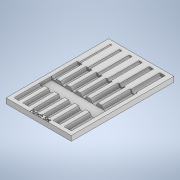
# Autodesk Inventor part: punchTray
Saved by Autodesk Inventor 2020.2 (Build 242310000, 310)
## iProperties
Created: 2019-12-07
Part Number: punchTray
Material: Generic
Document SubType Name: Modeling
Designer: robst
Density: 1 g/cm^3
Appearance: Default
Author: robst
Autodesk Inventor part; units mm, degrees
ref_plane "YZ Plane" through (0, 0, 0) normal (1, 0, 0) x (0, 1, 0)
ref_plane "XZ Plane" through (0, 0, 0) normal (0, 1, 0) x (-1, 0, 0)
ref_plane "XY Plane" through (0, 0, 0) normal (0, 0, 1) x (1, 0, 0)
sketch "Sketch3" plane through (0, 0, 0) normal (0, 0, 1) x (1, 0, 0)
  line L0 (-52.4636, -4.0957) -> (52.4636, -4.0957)
  line L1 (52.4636, -4.0957) -> (52.4636, 4.0958)
  line L2 (52.4636, 4.0958) -> (-52.4636, 4.0958)
  line L3 (-52.4636, 4.0958) -> (-52.4636, -4.0957)
  line L4 (-52.4636, -4.0957) -> (52.4636, 4.0958) construction
  line L5 (52.4636, -4.0957) -> (-52.4636, 4.0958) construction
  line L6 (46.1136, 4.0958) -> (43.2173, -0.9208)
  line L7 (43.2173, -0.9208) -> (37.4248, -0.9208)
  line L8 (37.4248, -0.9208) -> (34.5285, 4.0958)
  line L9 (34.5285, 4.0958) -> (37.4248, 9.1123)
  line L10 (37.4248, 9.1123) -> (43.2173, 9.1123)
  line L11 (43.2173, 9.1123) -> (46.1136, 4.0958)
  line L12 (28.1785, 4.0958) -> (25.2822, -0.9207)
  line L13 (25.2822, -0.9207) -> (19.4897, -0.9207)
  line L14 (19.4897, -0.9207) -> (16.5934, 4.0957)
  line L15 (16.5934, 4.0957) -> (19.4897, 9.1122)
  line L16 (19.4897, 9.1122) -> (25.2822, 9.1123)
  line L17 (25.2822, 9.1123) -> (28.1785, 4.0958)
  line L18 (0, 0) -> (0, 4.0957) construction
  line L19 (10.2434, 4.0958) -> (7.787, -0.1587)
  line L20 (7.787, -0.1587) -> (2.8744, -0.1587)
  line L21 (2.8744, -0.1587) -> (0.418, 4.0958)
  line L22 (0.418, 4.0958) -> (2.8744, 8.3503)
  line L23 (2.8744, 8.3503) -> (7.787, 8.3503)
  line L24 (7.787, 8.3503) -> (10.2434, 4.0958)
  line L25 (-5.932, 4.0958) -> (-8.3883, -0.1588)
  line L26 (-8.3883, -0.1588) -> (-13.301, -0.1587)
  line L27 (-13.301, -0.1587) -> (-15.7573, 4.0958)
  line L28 (-15.7573, 4.0958) -> (-13.301, 8.3503)
  line L29 (-13.301, 8.3503) -> (-8.3883, 8.3503)
  line L30 (-8.3883, 8.3503) -> (-5.932, 4.0958)
  line L31 (-22.1073, 4.0958) -> (-24.5416, -0.1206)
  line L32 (-24.5416, -0.1206) -> (-29.4103, -0.1206)
  line L33 (-29.4103, -0.1206) -> (-31.8447, 4.0958)
  line L34 (-31.8447, 4.0958) -> (-29.4103, 8.3122)
  line L35 (-29.4103, 8.3122) -> (-24.5416, 8.3122)
  line L36 (-24.5416, 8.3122) -> (-22.1073, 4.0958)
  line L37 (-38.1947, 4.0958) -> (-40.1744, 0.6668)
  line L38 (-40.1744, 0.6668) -> (-44.1339, 0.6668)
  line L39 (-44.1339, 0.6668) -> (-46.1136, 4.0958)
  line L40 (-46.1136, 4.0958) -> (-44.1339, 7.5248)
  line L41 (-44.1339, 7.5248) -> (-40.1744, 7.5247)
  line L42 (-40.1744, 7.5247) -> (-38.1947, 4.0958)
  point P0 (40.321, 4.0958)
  point P1 (22.3859, 4.0958)
  point P2 (34.5285, 4.0958)
  point P3 (16.5934, 4.0958)
  point P4 (5.3307, 4.0958)
  point P5 (-10.8446, 4.0958)
  point P6 (-26.976, 4.0958)
  point P7 (-42.1541, 4.0958)
  point P8 (0.418, 4.0958)
  point P9 (-15.7573, 4.0958)
  point P10 (-31.8447, 4.0958)
  point P11 (-46.1136, 4.0958)
  dimension "d7" = 10.033
  dimension "d8" = 10.033
  dimension "d13" = 6.35
  dimension "d14" = 6.35
  dimension "d15" = 8.509
  dimension "d16" = 6.35
  dimension "d17" = 8.509
  dimension "d18" = 6.35
  dimension "d19" = 8.4328
  dimension "d20" = 6.35
  dimension "d21" = 6.35
  dimension "d22" = 6.858
  dimension "d23" = 6.35
  dimension "d24" = 3.175
  constraints: 84 end point, 2 horizontal, 2 midpoint, 1 parallel, 1 perpendicular, 94 other
  measures "d7" distance between parallel lines of L7 L10
  measures "d8" distance between parallel lines of L13 L16
  measures "d13" distance of L6.start L1.end
  measures "d14" distance of L8.end L12.start
  measures "d15" distance between parallel lines of L20 L23
  measures "d16" distance of L14.end L19.start
  measures "d17" distance between parallel lines of L26 L29
  measures "d18" distance of L21.end L25.start
  measures "d19" distance between parallel lines of L32 L35
  measures "d20" distance of L27.end L31.start
  measures "d21" distance of L33.end L37.start
  measures "d22" distance between parallel lines of L38 L41
  measures "d23" distance from line of L39.end L3
  measures "d24" distance between parallel lines of L0 L7
extrude "Extrusion3" add sketch "Sketch3" against normal blind 152.4 contours L3 L2 L39 L38 L37 L33 L32 L31 L27 L26 L25 L21 L20 L19 L14 L13 L12 L8 L7 L6 L1 L0
sketch "Sketch4" plane through (0, 0, 0) normal (0, 0, 1) x (1, 0, 0)
  line L0 (52.4636, -4.0957) -> (-52.4636, -4.0957) projected
  line L1 (52.4636, 4.0958) -> (52.4636, -4.0957) projected
  line L2 (-52.4636, -4.0957) -> (52.4636, -4.0957)
  line L3 (52.4636, -4.0957) -> (52.4636, 4.0958)
  line L4 (52.4636, 4.0958) -> (-52.4636, 4.0957)
  line L5 (-52.4636, 4.0957) -> (-52.4636, -4.0957)
  point P0 (0, 0)
  constraints: 8 end point, 2 parallel, 1 horizontal, 1 perpendicular
extrude "Extrusion4" add sketch "Sketch4" along normal blind 6.35
sketch "Sketch6" plane through (0, 0, -152.4) normal (0, 0, -1) x (-1, 0, 0)
  line L0 (-37.4248, -0.9208) -> (-43.2173, -0.9208) construction
  line L1 (-40.321, -0.9208) -> (-40.321, 4.0958) construction
  line L2 (-52.4636, 4.0958) -> (52.4636, 4.0957) construction
  arc A0 (-44.5438, 4.0958) -> (-36.0983, 4.0958) centre (-40.321, 4.0958) ccw
  line L3 (-34.5285, 4.0958) -> (-37.4248, -0.9208)
  line L4 (-37.4248, -0.9208) -> (-43.2173, -0.9208)
  line L5 (-43.2173, -0.9208) -> (-46.1136, 4.0958)
  line L6 (-46.1136, 4.0958) -> (-44.5438, 4.0958)
  line L7 (-34.5285, 4.0958) -> (-36.0983, 4.0958)
  point P0 (0, 0)
  dimension "d31" = 8.4455
  constraints: 12 end point, 3 point on line, 2 coincident, 2 point on circle, 1 centre point, 1 midpoint, 1 vertical, 6 other
  measures "d31" diameter of A0
extrude "5_16_punch" add sketch "Sketch6" against normal blind 46.355
sketch "Sketch7" plane through (0, 0, -152.4) normal (0, 0, -1) x (-1, 0, 0)
  line L0 (-28.1785, 4.0958) -> (-16.5934, 4.0958) projected
  line L1 (-16.5934, 4.0958) -> (-19.4897, -0.9207)
  line L2 (-19.4897, -0.9207) -> (-25.2822, -0.9207)
  line L3 (-25.2822, -0.9207) -> (-28.1785, 4.0958)
  arc A0 (-25.8149, 4.0958) -> (-18.9569, 4.0958) centre (-22.3859, 4.0958) ccw
  line L4 (-28.1785, 4.0958) -> (-25.8149, 4.0958)
  line L5 (-10.2434, 4.0958) -> (-16.5934, 4.0958) projected
  line L6 (-16.5934, 4.0958) -> (-18.9569, 4.0958)
  point P0 (0, 0)
  dimension "d34" = 6.858
  constraints: 10 end point, 2 point on circle, 2 point on line, 1 centre point, 1 coincident, 1 midpoint, 6 other
  measures "d34" diameter of A0
extrude "1_4_punch" add sketch "Sketch7" against normal blind 47.625 contours L0 A0 L1 L2 L3
sketch "Sketch8" plane through (0, 0, -152.4) normal (0, 0, -1) x (-1, 0, 0)
  line L0 (-10.2434, 4.0958) -> (-0.418, 4.0958) projected
  line L1 (-0.418, 4.0958) -> (-2.8744, -0.1588)
  line L2 (-2.8744, -0.1588) -> (-7.787, -0.1587)
  line L3 (-7.787, -0.1587) -> (-10.2434, 4.0958)
  arc A0 (-7.966, 4.0958) -> (-2.6955, 4.0958) centre (-5.3307, 4.0958) ccw
  line L4 (-10.2434, 4.0958) -> (-7.787, -0.1587) projected
  line L5 (-10.2434, 4.0958) -> (-7.966, 4.0958)
  line L6 (-0.418, 4.0958) -> (-2.6955, 4.0958)
  point P0 (0, 0)
  point P1 (-10.2434, 4.0958)
  dimension "d37" = 5.2705
  constraints: 10 end point, 2 point on circle, 2 point on line, 1 centre point, 1 coincident, 1 midpoint, 6 other
  measures "d37" diameter of A0
extrude "3_16_punch" add sketch "Sketch8" against normal blind 50.8 contours L0 A0 L1 L2 L3
sketch "Sketch9" plane through (0, 0, -152.4) normal (0, 0, -1) x (-1, 0, 0)
  line L0 (13.301, -0.1587) -> (8.3883, -0.1588) construction
  line L1 (10.8446, -0.1587) -> (10.8446, 4.0957) construction
  line L2 (-52.4636, 4.0958) -> (52.4636, 4.0957) construction
  line L3 (15.7573, 4.0958) -> (13.301, -0.1587) projected
  line L4 (15.7573, 4.0958) -> (13.301, -0.1588)
  line L5 (13.301, -0.1588) -> (8.3883, -0.1588)
  line L6 (8.3883, -0.1588) -> (5.932, 4.0958)
  arc A0 (8.6063, 4.0957) -> (13.083, 4.0957) centre (10.8446, 4.0957) ccw
  line L7 (8.3883, -0.1588) -> (5.932, 4.0958) projected
  line L8 (5.932, 4.0958) -> (8.6063, 4.0957)
  line L9 (22.1073, 4.0958) -> (15.7573, 4.0958) projected
  line L10 (15.7573, 4.0958) -> (13.083, 4.0957)
  point P0 (0, 0)
  point P1 (13.301, -0.1588)
  dimension "d40" = 4.4768
  constraints: 12 end point, 3 point on line, 2 coincident, 2 point on circle, 1 centre point, 1 midpoint, 1 vertical, 6 other
  measures "d40" diameter of A0
extrude "5_32_punch" add sketch "Sketch9" against normal blind 50.8
sketch "Sketch11" plane through (0, 0, -152.4) normal (0, 0, -1) x (-1, 0, 0)
  line L0 (22.1073, 4.0958) -> (31.8447, 4.0958) projected
  line L1 (29.4103, -0.1206) -> (31.8447, 4.0958) projected
  line L2 (31.8447, 4.0958) -> (29.4103, -0.1206)
  line L3 (29.4103, -0.1206) -> (24.5416, -0.1206)
  line L4 (24.5416, -0.1206) -> (22.1073, 4.0958)
  arc A0 (25.1345, 4.0958) -> (28.8175, 4.0958) centre (26.976, 4.0958) ccw
  line L5 (22.1073, 4.0958) -> (24.5416, -0.1206) projected
  line L6 (22.1073, 4.0958) -> (25.1345, 4.0958)
  line L7 (31.8447, 4.0958) -> (28.8175, 4.0958)
  point P0 (0, 0)
  point P1 (29.4103, -0.1206)
  dimension "d44" = 3.683
  constraints: 10 end point, 2 point on circle, 2 point on line, 1 centre point, 1 coincident, 1 midpoint, 6 other
  measures "d44" diameter of A0
extrude "1_8_punch" add sketch "Sketch11" against normal blind 50.8 contours L0 A0 L1 L3 L4
sketch "Sketch12" plane through (0, 0, -152.4) normal (0, 0, -1) x (-1, 0, 0)
  line L0 (40.1744, 0.6668) -> (44.1339, 0.6668) construction
  line L1 (42.1541, 0.6668) -> (42.1541, 4.0957) construction
  line L2 (-52.4636, 4.0958) -> (52.4636, 4.0957) construction
  line L3 (44.1339, 0.6668) -> (46.1136, 4.0958) projected
  line L4 (46.1136, 4.0958) -> (44.1339, 0.6668)
  line L5 (44.1339, 0.6668) -> (40.1744, 0.6667)
  line L6 (40.1744, 0.6667) -> (38.1947, 4.0958)
  arc A0 (41.1064, 4.0957) -> (43.2019, 4.0957) centre (42.1541, 4.0957) ccw
  line L7 (38.1947, 4.0958) -> (28.8175, 4.0958) projected
  line L8 (38.1947, 4.0958) -> (41.1064, 4.0957)
  line L9 (46.1136, 4.0958) -> (43.2019, 4.0957)
  point P0 (0, 0)
  point P1 (44.1339, 0.6668)
  dimension "d47" = 2.0955
  constraints: 12 end point, 3 point on line, 2 coincident, 2 point on circle, 1 centre point, 1 midpoint, 1 vertical, 6 other
  measures "d47" diameter of A0
extrude "1_16_punch" add sketch "Sketch12" against normal blind 50.8
sketch "Sketch5" plane through (0, 0, -152.4) normal (0, 0, -1) x (-1, 0, 0)
  line L0 (-52.4636, 4.0958) -> (-52.4636, -4.0957) projected
  line L1 (52.4636, 4.0958) -> (46.1136, 4.0958) projected
  line L2 (-52.4636, -4.0957) -> (52.4636, -4.0957)
  line L3 (52.4636, -4.0957) -> (52.4636, 4.0958)
  line L4 (52.4636, 4.0958) -> (-52.4636, 4.0957)
  line L5 (-52.4636, 4.0957) -> (-52.4636, -4.0957)
  point P0 (0, 0)
  point P1 (-52.4636, 4.0957)
  constraints: 8 end point, 2 parallel, 1 horizontal, 1 perpendicular
extrude "Extrusion5" add sketch "Sketch5" along normal blind 6.35
sketch "Sketch13" plane through (-52.4636, 4.0958, 6.35) normal (0, 1, 0) x (1, 0, 0)
  line L0 (6.35, 6.35) -> (6.35, 107.95) projected
  line L1 (98.5772, 6.35) -> (98.5772, 112.395) projected
  line L2 (6.35, 47.625) -> (98.5772, 47.625)
  line L3 (98.5772, 47.625) -> (98.5772, 66.675)
  line L4 (98.5772, 66.675) -> (6.35, 66.675)
  line L5 (6.35, 66.675) -> (6.35, 47.625)
  line L6 (6.35, 57.15) -> (98.5772, 57.15) construction
  line L7 (14.2689, 6.35) -> (6.35, 6.35) construction
  point P0 (52.4636, 6.35)
  point P1 (6.35, 66.675)
  dimension "d50" = 19.05
  dimension "d51" = 50.8
  constraints: 10 end point, 2 midpoint, 2 parallel, 2 point on line, 1 horizontal, 1 perpendicular
  measures "d50" distance between parallel lines of L4 L2
  measures "d51" distance between parallel lines of L6 L7
extrude "Extrusion12" cut sketch "Sketch13" against normal blind 5.08
sketch "Sketch14" plane through (-52.4636, 4.0958, 6.35) normal (0, 1, 0) x (1, 0, 0)
  line L0 (0, 165.1) -> (0, 0) construction
  line L1 (0, 3.175) -> (104.9272, 3.175) construction
  line L2 (0, 0) -> (104.9272, 0) construction
  spline S0 degree 2 poles (40.766, 4.1836) (40.766, 3.8543) (40.5314, 3.2615) (40.3214, 3.0556) knots 0 0 0 1 2 2 2
  spline S1 degree 2 poles (40.3214, 3.0556) (40.0579, 2.7963) (39.3458, 2.5287) (38.8024, 2.5287) knots 0 0 0 1 2 2 2
  line L3 (38.8024, 2.5287) -> (38.2301, 2.5287)
  line L4 (38.2301, 2.5287) -> (38.2301, 0.635)
  line L5 (38.2301, 0.635) -> (37.555, 0.635)
  line L6 (37.555, 0.635) -> (37.555, 5.715)
  line L7 (37.555, 5.715) -> (38.8312, 5.715)
  spline S2 degree 2 poles (38.8312, 5.715) (39.284, 5.715) (39.918, 5.5668) (40.1609, 5.398) knots 0 0 0 1 2 2 2
  spline S3 degree 2 poles (40.1609, 5.398) (40.4449, 5.2045) (40.766, 4.6076) (40.766, 4.1836) knots 0 0 0 1 2 2 2
  spline S4 degree 2 poles (40.0621, 4.163) (40.0621, 4.4265) (39.8809, 4.8134) (39.6957, 4.9369) knots 0 0 0 1 2 2 2
  spline S5 degree 2 poles (39.6957, 4.9369) (39.5351, 5.044) (39.107, 5.1304) (38.79, 5.1304) knots 0 0 0 1 2 2 2
  line L8 (38.79, 5.1304) -> (38.2301, 5.1304)
  line L9 (38.2301, 5.1304) -> (38.2301, 3.105)
  line L10 (38.2301, 3.105) -> (38.6912, 3.105)
  spline S6 degree 2 poles (38.6912, 3.105) (39.1029, 3.105) (39.6092, 3.2368) (39.7739, 3.4097) knots 0 0 0 1 2 2 2
  spline S7 degree 2 poles (39.7739, 3.4097) (39.9262, 3.562) (40.0621, 3.9201) (40.0621, 4.163) knots 0 0 0 1 2 2 2
  line L11 (44.3228, 0.635) -> (43.6806, 0.635)
  line L12 (43.6806, 0.635) -> (43.6806, 1.0549)
  spline S8 degree 2 poles (43.6806, 1.0549) (43.3842, 0.7956) (42.8532, 0.528) (42.5238, 0.528) knots 0 0 0 1 2 2 2
  spline S9 degree 2 poles (42.5238, 0.528) (42.2768, 0.528) (41.8364, 0.6926) (41.6758, 0.8697) knots 0 0 0 1 2 2 2
  spline S10 degree 2 poles (41.6758, 0.8697) (41.5111, 1.0467) (41.33, 1.586) (41.33, 1.9729) knots 0 0 0 1 2 2 2
  line L13 (41.33, 1.9729) -> (41.33, 4.4471)
  line L14 (41.33, 4.4471) -> (41.9722, 4.4471)
  line L15 (41.9722, 4.4471) -> (41.9722, 2.2734)
  spline S11 degree 2 poles (41.9722, 2.2734) (41.9722, 1.9688) (42.0175, 1.5695) (42.0957, 1.4213) knots 0 0 0 1 2 2 2
  spline S12 degree 2 poles (42.0957, 1.4213) (42.1739, 1.2731) (42.4415, 1.1372) (42.6926, 1.1372) knots 0 0 0 1 2 2 2
  spline S13 degree 2 poles (42.6926, 1.1372) (42.9273, 1.1372) (43.4583, 1.4048) (43.6806, 1.5983) knots 0 0 0 1 2 2 2
  line L16 (43.6806, 1.5983) -> (43.6806, 4.4471)
  line L17 (43.6806, 4.4471) -> (44.3228, 4.4471)
  line L18 (44.3228, 4.4471) -> (44.3228, 0.635)
  line L19 (48.2461, 0.635) -> (47.6038, 0.635)
  line L20 (47.6038, 0.635) -> (47.6038, 2.8086)
  spline S14 degree 2 poles (47.6038, 2.8086) (47.6038, 3.0721) (47.5544, 3.5249) (47.4803, 3.6608) knots 0 0 0 1 2 2 2
  spline S15 degree 2 poles (47.4803, 3.6608) (47.4021, 3.8049) (47.1222, 3.9448) (46.8834, 3.9448) knots 0 0 0 1 2 2 2
  spline S16 degree 2 poles (46.8834, 3.9448) (46.6447, 3.9448) (46.1383, 3.6896) (45.8954, 3.4838) knots 0 0 0 1 2 2 2
  line L21 (45.8954, 3.4838) -> (45.8954, 0.635)
  line L22 (45.8954, 0.635) -> (45.2532, 0.635)
  line L23 (45.2532, 0.635) -> (45.2532, 4.4471)
  line L24 (45.2532, 4.4471) -> (45.8954, 4.4471)
  line L25 (45.8954, 4.4471) -> (45.8954, 4.023)
  spline S17 degree 2 poles (45.8954, 4.023) (46.1836, 4.2824) (46.7393, 4.5541) (47.0522, 4.5541) knots 0 0 0 1 2 2 2
  spline S18 degree 2 poles (47.0522, 4.5541) (47.6121, 4.5541) (48.2461, 3.8131) (48.2461, 3.1091) knots 0 0 0 1 2 2 2
  line L26 (48.2461, 3.1091) -> (48.2461, 0.635)
  spline S19 degree 2 poles (50.6626, 0.5485) (50.2673, 0.5485) (49.6128, 0.7914) (49.3781, 1.0384) knots 0 0 0 1 2 2 2
  spline S20 degree 2 poles (49.3781, 1.0384) (49.1435, 1.2813) (48.8841, 2.0306) (48.8841, 2.5328) knots 0 0 0 1 2 2 2
  spline S21 degree 2 poles (48.8841, 2.5328) (48.8841, 3.035) (49.1517, 3.7678) (49.3781, 4.0148) knots 0 0 0 1 2 2 2
  spline S22 degree 2 poles (49.3781, 4.0148) (49.6046, 4.2659) (50.2756, 4.5335) (50.6626, 4.5335) knots 0 0 0 1 2 2 2
  spline S23 degree 2 poles (50.6626, 4.5335) (50.9754, 4.5335) (51.56, 4.3565) (51.7864, 4.2412) knots 0 0 0 1 2 2 2
  line L27 (51.7864, 4.2412) -> (51.7864, 3.5208)
  line L28 (51.7864, 3.5208) -> (51.7494, 3.5208)
  spline S24 degree 2 poles (51.7494, 3.5208) (51.6794, 3.5784) (51.4653, 3.7266) (51.313, 3.8049) knots 0 0 0 1 2 2 2
  spline S25 degree 2 poles (51.313, 3.8049) (51.1771, 3.8707) (50.8149, 3.9736) (50.6502, 3.9736) knots 0 0 0 1 2 2 2
  spline S26 degree 2 poles (50.6502, 3.9736) (50.1521, 3.9736) (49.5469, 3.2203) (49.5469, 2.5328) knots 0 0 0 1 2 2 2
  spline S27 degree 2 poles (49.5469, 2.5328) (49.5469, 1.8618) (50.1315, 1.1084) (50.6502, 1.1084) knots 0 0 0 1 2 2 2
  spline S28 degree 2 poles (50.6502, 1.1084) (50.9631, 1.1084) (51.5312, 1.3678) (51.7494, 1.5695) knots 0 0 0 1 2 2 2
  line L29 (51.7494, 1.5695) -> (51.7864, 1.5695)
  line L30 (51.7864, 1.5695) -> (51.7864, 0.8491)
  spline S29 degree 2 poles (51.7864, 0.8491) (51.6917, 0.8038) (51.4036, 0.6762) (51.2883, 0.6474) knots 0 0 0 1 2 2 2
  spline S30 degree 2 poles (51.2883, 0.6474) (51.1236, 0.5979) (50.8643, 0.5485) (50.6626, 0.5485) knots 0 0 0 1 2 2 2
  line L31 (55.3638, 0.635) -> (54.7216, 0.635)
  line L32 (54.7216, 0.635) -> (54.7216, 2.8086)
  spline S31 degree 2 poles (54.7216, 2.8086) (54.7216, 3.0721) (54.6722, 3.5249) (54.5981, 3.6608) knots 0 0 0 1 2 2 2
  spline S32 degree 2 poles (54.5981, 3.6608) (54.5199, 3.8049) (54.24, 3.9448) (54.0012, 3.9448) knots 0 0 0 1 2 2 2
  spline S33 degree 2 poles (54.0012, 3.9448) (53.7624, 3.9448) (53.2561, 3.6896) (53.0132, 3.4838) knots 0 0 0 1 2 2 2
  line L33 (53.0132, 3.4838) -> (53.0132, 0.635)
  line L34 (53.0132, 0.635) -> (52.371, 0.635)
  line L35 (52.371, 0.635) -> (52.371, 5.9414)
  line L36 (52.371, 5.9414) -> (53.0132, 5.9414)
  line L37 (53.0132, 5.9414) -> (53.0132, 4.023)
  spline S34 degree 2 poles (53.0132, 4.023) (53.3014, 4.2824) (53.8571, 4.5541) (54.17, 4.5541) knots 0 0 0 1 2 2 2
  spline S35 degree 2 poles (54.17, 4.5541) (54.7298, 4.5541) (55.3638, 3.8131) (55.3638, 3.1091) knots 0 0 0 1 2 2 2
  line L38 (55.3638, 3.1091) -> (55.3638, 0.635)
  spline S36 degree 2 poles (59.9128, 0.5444) (59.3611, 0.5444) (58.5872, 0.775) (58.2455, 0.9396) knots 0 0 0 1 2 2 2
  line L39 (58.2455, 0.9396) -> (58.2455, 1.7877)
  line L40 (58.2455, 1.7877) -> (58.2949, 1.7877)
  spline S37 degree 2 poles (58.2949, 1.7877) (58.6284, 1.4748) (59.4723, 1.129) (59.8634, 1.129) knots 0 0 0 1 2 2 2
  spline S38 degree 2 poles (59.8634, 1.129) (60.4232, 1.129) (60.9955, 1.5942) (60.9955, 1.977) knots 0 0 0 1 2 2 2
  spline S39 degree 2 poles (60.9955, 1.977) (60.9955, 2.2817) (60.6949, 2.6604) (60.3697, 2.7551) knots 0 0 0 1 2 2 2
  spline S40 degree 2 poles (60.3697, 2.7551) (60.1351, 2.821) (59.744, 2.9115) (59.4517, 2.9856) knots 0 0 0 1 2 2 2
  spline S41 degree 2 poles (59.4517, 2.9856) (59.1882, 3.0556) (58.7724, 3.2656) (58.6119, 3.4344) knots 0 0 0 1 2 2 2
  spline S42 degree 2 poles (58.6119, 3.4344) (58.4555, 3.6031) (58.2826, 4.056) (58.2826, 4.3524) knots 0 0 0 1 2 2 2
  spline S43 degree 2 poles (58.2826, 4.3524) (58.2826, 4.9699) (59.2459, 5.8056) (59.991, 5.8056) knots 0 0 0 1 2 2 2
  spline S44 degree 2 poles (59.991, 5.8056) (60.4191, 5.8056) (61.1766, 5.6368) (61.5018, 5.4762) knots 0 0 0 1 2 2 2
  line L41 (61.5018, 5.4762) -> (61.5018, 4.6694)
  line L42 (61.5018, 4.6694) -> (61.4524, 4.6694)
  spline S45 degree 2 poles (61.4524, 4.6694) (61.2095, 4.8917) (60.452, 5.221) (60.0363, 5.221) knots 0 0 0 1 2 2 2
  spline S46 degree 2 poles (60.0363, 5.221) (59.567, 5.221) (58.9865, 4.7805) (58.9865, 4.4224) knots 0 0 0 1 2 2 2
  spline S47 degree 2 poles (58.9865, 4.4224) (58.9865, 4.1013) (59.3282, 3.7184) (59.6493, 3.632) knots 0 0 0 1 2 2 2
  spline S48 degree 2 poles (59.6493, 3.632) (59.8634, 3.5743) (60.485, 3.4261) (60.6908, 3.3644) knots 0 0 0 1 2 2 2
  spline S49 degree 2 poles (60.6908, 3.3644) (61.2136, 3.2038) (61.6994, 2.5575) (61.6994, 2.0841) knots 0 0 0 1 2 2 2
  spline S50 degree 2 poles (61.6994, 2.0841) (61.6994, 1.7836) (61.4565, 1.2072) (61.2383, 1.0055) knots 0 0 0 1 2 2 2
  spline S51 degree 2 poles (61.2383, 1.0055) (60.9955, 0.7832) (60.3779, 0.5444) (59.9128, 0.5444) knots 0 0 0 1 2 2 2
  spline S52 degree 2 poles (63.9924, 0.5485) (63.0785, 0.5485) (62.074, 1.5736) (62.074, 2.5204) knots 0 0 0 1 2 2 2
  spline S53 degree 2 poles (62.074, 2.5204) (62.074, 3.4508) (63.0497, 4.5541) (63.836, 4.5541) knots 0 0 0 1 2 2 2
  spline S54 degree 2 poles (63.836, 4.5541) (64.19, 4.5541) (64.7375, 4.3483) (64.9392, 4.1301) knots 0 0 0 1 2 2 2
  spline S55 degree 2 poles (64.9392, 4.1301) (65.1451, 3.9119) (65.3633, 3.282) (65.3633, 2.8251) knots 0 0 0 1 2 2 2
  line L43 (65.3633, 2.8251) -> (65.3633, 2.4752)
  line L44 (65.3633, 2.4752) -> (62.7245, 2.4752)
  spline S56 degree 2 poles (62.7245, 2.4752) (62.7245, 1.8124) (63.3914, 1.1084) (63.9842, 1.1084) knots 0 0 0 1 2 2 2
  spline S57 degree 2 poles (63.9842, 1.1084) (64.1941, 1.1084) (64.6017, 1.2031) (64.7663, 1.2772) knots 0 0 0 1 2 2 2
  spline S58 degree 2 poles (64.7663, 1.2772) (64.9392, 1.3595) (65.178, 1.5036) (65.2562, 1.5695) knots 0 0 0 1 2 2 2
  line L45 (65.2562, 1.5695) -> (65.2933, 1.5695)
  line L46 (65.2933, 1.5695) -> (65.2933, 0.8697)
  spline S59 degree 2 poles (65.2933, 0.8697) (65.1821, 0.8244) (64.8446, 0.6926) (64.7128, 0.6556) knots 0 0 0 1 2 2 2
  spline S60 degree 2 poles (64.7128, 0.6556) (64.5276, 0.6021) (64.2229, 0.5485) (63.9924, 0.5485) knots 0 0 0 1 2 2 2
  spline S61 degree 2 poles (64.7375, 2.965) (64.7293, 3.2244) (64.6223, 3.6031) (64.5193, 3.7308) knots 0 0 0 1 2 2 2
  spline S62 degree 2 poles (64.5193, 3.7308) (64.4082, 3.8748) (64.0583, 4.0272) (63.7989, 4.0272) knots 0 0 0 1 2 2 2
  spline S63 degree 2 poles (63.7989, 4.0272) (63.5437, 4.0272) (63.1855, 3.8748) (63.0373, 3.7266) knots 0 0 0 1 2 2 2
  spline S64 degree 2 poles (63.0373, 3.7266) (62.8932, 3.5743) (62.745, 3.2079) (62.7245, 2.965) knots 0 0 0 1 2 2 2
  line L47 (62.7245, 2.965) -> (64.7375, 2.965)
  spline S65 degree 2 poles (67.1664, 0.5609) (66.6436, 0.5609) (66.0549, 1.1578) (66.0549, 1.8041) knots 0 0 0 1 2 2 2
  line L48 (66.0549, 1.8041) -> (66.0549, 3.916)
  line L49 (66.0549, 3.916) -> (65.6226, 3.916)
  line L50 (65.6226, 3.916) -> (65.6226, 4.4471)
  line L51 (65.6226, 4.4471) -> (66.0549, 4.4471)
  line L52 (66.0549, 4.4471) -> (66.0549, 5.5421)
  line L53 (66.0549, 5.5421) -> (66.6971, 5.5421)
  line L54 (66.6971, 5.5421) -> (66.6971, 4.4471)
  line L55 (66.6971, 4.4471) -> (67.8786, 4.4471)
  line L56 (67.8786, 4.4471) -> (67.8786, 3.916)
  line L57 (67.8786, 3.916) -> (66.6971, 3.916)
  line L58 (66.6971, 3.916) -> (66.6971, 2.1005)
  spline S66 degree 2 poles (66.6971, 2.1005) (66.6971, 1.8124) (66.7177, 1.4954) (66.7876, 1.3595) knots 0 0 0 1 2 2 2
  spline S67 degree 2 poles (66.7876, 1.3595) (66.8453, 1.2402) (67.1046, 1.1208) (67.3269, 1.1208) knots 0 0 0 1 2 2 2
  spline S68 degree 2 poles (67.3269, 1.1208) (67.4834, 1.1208) (67.7756, 1.2155) (67.8415, 1.2443) knots 0 0 0 1 2 2 2
  line L59 (67.8415, 1.2443) -> (67.8786, 1.2443)
  line L60 (67.8786, 1.2443) -> (67.8786, 0.6679)
  spline S69 degree 2 poles (67.8786, 0.6679) (67.6974, 0.6185) (67.3269, 0.5609) (67.1664, 0.5609) knots 0 0 0 1 2 2 2
  point P0 (52.4636, 6.35)
  dimension "d54" = 3.175
  constraints: 2 end point, 1 horizontal, 1 parallel, 1 point on line
  measures "d54" distance between parallel lines of L1 L2
extrude "Extrusion13" cut sketch "Sketch14" against normal blind 3.175
equation "\"d14\" = gapBetweenParts"
equation "\"d16\" = gapBetweenParts"
equation "\"d18\" = gapBetweenParts"
equation "\"d20\" = gapBetweenParts"
equation "\"d21\" = gapBetweenParts"
equation "\"gapBetweenParts\" = 6.35"
body "Solid3"
